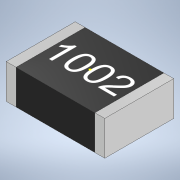
# Autodesk Inventor part: Part4
Saved by Autodesk Inventor 2021 (Build 250183000, 183)
## iProperties
Created: 2023-04-01
Part Number: Part4
Material: Generic
Document SubType Name: Modeling
Designer: stepa
Density: 1 g/cm^3
Appearance: Default
Author: stepa
Autodesk Inventor part; units mm, degrees
ref_plane "YZ Plane" through (0, 0, 0) normal (1, 0, 0) x (0, 1, 0)
ref_plane "XZ Plane" through (0, 0, 0) normal (0, 1, 0) x (-1, 0, 0)
ref_plane "XY Plane" through (0, 0, 0) normal (0, 0, 1) x (1, 0, 0)
sketch "Sketch1" plane through (0, 0, 0) normal (0, 1, 0) x (-1, 0, 0)
  line L0 (0.8, 0.7) -> (-0.8, 0.7)
  line L1 (-0.8, 0.7) -> (-0.8, -0.7)
  line L2 (-0.8, -0.7) -> (0.8, -0.7)
  line L3 (0.8, -0.7) -> (0.8, 0.7)
  line L4 (0.8, 0.7) -> (-0.8, -0.7) construction
  line L5 (-0.8, 0.7) -> (0.8, -0.7) construction
  point P0 (0, 0)
  dimension "d0" = 1.4
  dimension "d1" = 1.6
  constraints: 12 end point, 2 midpoint, 2 parallel, 1 horizontal, 1 perpendicular
  measures "d0" distance of L2.end L0.start
  measures "d1" distance of L1.end L2.end
extrude "Extrusion1" add sketch "Sketch1" along normal blind 0.7
sketch "Sketch2" plane through (0.8, 0, 0.7) normal (1, 0, 0) x (0, 0, -1)
  line L0 (0, 0) -> (1.4, 0) projected
  line L1 (1.4, 0) -> (1.4, 0.7) projected
  line L2 (0, 0.7) -> (1.4, 0.7) projected
  line L3 (0, 0) -> (0, 0.7) projected
  point P0 (0.7, 0)
extrude "Extrusion2" add sketch "Sketch2" along normal blind 0.2 separate body
mirror "Mirror1" about plane through (0, 0, 0) normal (1, 0, 0) of "Extrusion2" bodies 2
sketch "Sketch3" plane through (0, 0.7, 0) normal (0, 1, 0) x (1, 0, 0)
  line L0 (-0.809, 0.2813) -> (2.4608, 0.2813) construction
  line L1 (2.4608, 0.2813) -> (2.4608, -0.6207) construction
  line L2 (2.4608, -0.6207) -> (-0.809, -0.6207) construction
  line L3 (-0.809, -0.6207) -> (-0.809, 0.2813) construction
  point P0 (0, 0)
  constraints: 2 other
body "Solid1"
body "Solid2"
